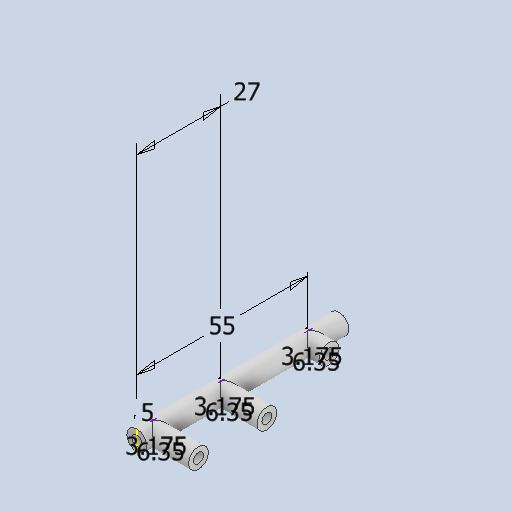
# Autodesk Inventor part: Valve Tube
Saved by Autodesk Inventor 2023 (Build 270158000, 158)
## iProperties
Created: 2024-03-20
Part Number: Valve Tube
Material: Generic
Document SubType Name: Modeling
Designer: Pobe Tran
Density: 1 g/cm^3
Appearance: Default
Author: Pobe Tran
Autodesk Inventor part; units mm, degrees
ref_plane "YZ Plane" through (0, 0, 0) normal (1, 0, 0) x (0, 1, 0)
ref_plane "XZ Plane" through (0, 0, 0) normal (0, 1, 0) x (-1, 0, 0)
ref_plane "XY Plane" through (0, 0, 0) normal (0, 0, 1) x (1, 0, 0)
sketch "Sketch1" plane through (0, 0, 0) normal (0, 0, 1) x (1, 0, 0)
  circle A0 centre (0, 0) radius 3.175
  circle A1 centre (0, 0) radius 1.5875
  dimension "d0" = 6.35
  dimension "d1" = 3.175
  constraints: 2 centre point, 2 coincident
  measures "d0" diameter of A0
  measures "d1" diameter of A1
extrude "Extrusion1" add sketch "Sketch1" along normal blind 65
sketch "Sketch2" plane through (0, 0, 0) normal (1, 0, 0) x (0, 1, 0)
  circle A0 centre (0, 60) radius 3.175
  circle A1 centre (0, 60) radius 1.5875
  line L0 (3.175, 65) -> (-3.175, 65) projected
  circle A2 centre (0, 38) radius 3.175
  circle A3 centre (0, 38) radius 1.5875
  circle A4 centre (0, 10) radius 3.175
  circle A5 centre (0, 10) radius 1.5875
  point P0 (0, 0)
  dimension "d4" = 6.35
  dimension "d5" = 3.175
  dimension "d6" = 5
  dimension "d7" = 6.35
  dimension "d8" = 3.175
  dimension "d9" = 27
  dimension "d10" = 6.35
  dimension "d11" = 3.175
  dimension "d12" = 55
  constraints: 6 centre point, 3 coincident, 2 vertical alignment
  measures "d4" diameter of A0
  measures "d5" diameter of A1
  measures "d6" distance from line of A0.centre L0
  measures "d7" diameter of A2
  measures "d8" diameter of A3
  measures "d9" distance from line of L0 A2.centre
  measures "d10" diameter of A4
  measures "d11" diameter of A5
  measures "d12" distance from line of A4.centre L0
extrude "Extrusion2" add sketch "Sketch2" along normal blind 14.825 contours A0 | A2
extrude "Extrusion3" add sketch "Sketch2" along normal blind 6.825 contours A4
body "Solid1"
